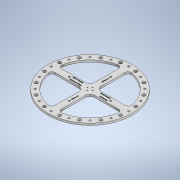
# Autodesk Inventor part: 24_Disco
Saved by Autodesk Inventor 2020.2 (Build 242310000, 310)
## iProperties
Created: 2019-11-29
Part Number: 24_Disco
Material: Generico
Document SubType Name: Modeling
Designer: socci
Density: 1 g/cm^3
Appearance: Default
Author: socci
Autodesk Inventor part; units mm, degrees
(part 1 of 3)
ref_plane "YZ Plane" through (0, 0, 0) normal (1, 0, 0) x (0, 1, 0)
ref_plane "XZ Plane" through (0, 0, 0) normal (0, 1, 0) x (-1, 0, 0)
ref_plane "XY Plane" through (0, 0, 0) normal (0, 0, 1) x (1, 0, 0)
sketch "Schizzo1" plane through (0, 0, 0) normal (0, 1, 0) x (-1, 0, 0)
  circle A0 centre (0, 0) radius 130
  line L0 (0, 130) -> (0, -130)
  line L1 (130, 0) -> (-130, 0)
  line L2 (10, 97.9796) -> (10, 23.6854)
  line L3 (97.9796, 10) -> (23.6854, 10)
  arc A1 (16.045, 13.5484) -> (13.5484, 16.045) centre (0, 0) ccw
  arc A2 (107.7775, 22) -> (22, 107.7775) centre (0, 0) ccw
  arc A3 (22, 107.7775) -> (10, 97.9796) centre (20, 97.9796) ccw
  arc A4 (10, 23.6854) -> (13.5484, 16.045) centre (20, 23.6854) ccw
  arc A5 (16.045, 13.5484) -> (23.6854, 10) centre (23.6854, 20) ccw
  arc A6 (97.9796, 10) -> (107.7775, 22) centre (97.9796, 20) ccw
  arc A7 (-13.5484, 16.045) -> (-10, 23.6854) centre (-20, 23.6854) ccw
  arc A8 (-13.5484, 16.045) -> (-16.045, 13.5484) centre (0, 0) ccw
  arc A9 (-23.6854, 10) -> (-16.045, 13.5484) centre (-23.6854, 20) ccw
  line L4 (-10, 97.9796) -> (-10, 23.6854)
  line L5 (-97.9796, 10) -> (-23.6854, 10)
  arc A10 (-107.7775, 22) -> (-97.9796, 10) centre (-97.9796, 20) ccw
  arc A11 (-22, 107.7775) -> (-107.7775, 22) centre (0, 0) ccw
  arc A12 (-10, 97.9796) -> (-22, 107.7775) centre (-20, 97.9796) ccw
  arc A13 (-16.045, -13.5484) -> (-23.6854, -10) centre (-23.6854, -20) ccw
  arc A14 (-16.045, -13.5484) -> (-13.5484, -16.045) centre (0, 0) ccw
  arc A15 (-10, -23.6854) -> (-13.5484, -16.045) centre (-20, -23.6854) ccw
  line L6 (-97.9796, -10) -> (-23.6854, -10)
  line L7 (-10, -97.9796) -> (-10, -23.6854)
  arc A16 (-22, -107.7775) -> (-10, -97.9796) centre (-20, -97.9796) ccw
  arc A17 (-107.7775, -22) -> (-22, -107.7775) centre (0, 0) ccw
  arc A18 (-97.9796, -10) -> (-107.7775, -22) centre (-97.9796, -20) ccw
  arc A19 (13.5484, -16.045) -> (10, -23.6854) centre (20, -23.6854) ccw
  arc A20 (13.5484, -16.045) -> (16.045, -13.5484) centre (0, 0) ccw
  arc A21 (23.6854, -10) -> (16.045, -13.5484) centre (23.6854, -20) ccw
  line L8 (10, -97.9796) -> (10, -23.6854)
  line L9 (97.9796, -10) -> (23.6854, -10)
  arc A22 (107.7775, -22) -> (97.9796, -10) centre (97.9796, -20) ccw
  arc A23 (22, -107.7775) -> (107.7775, -22) centre (0, 0) ccw
  arc A24 (10, -97.9796) -> (22, -107.7775) centre (20, -97.9796) ccw
  point P0 (18.4662, 10)
  point P1 (10, 18.4662)
  point P2 (109.5445, 10)
  point P3 (10, 109.5445)
  point P4 (-10, 18.4662)
  point P5 (-18.4662, 10)
  point P6 (-10, 109.5445)
  point P7 (-109.5445, 10)
  point P8 (-18.4662, -10)
  point P9 (-10, -18.4662)
  point P10 (-109.5445, -10)
  point P11 (-10, -109.5445)
  point P12 (10, -18.4662)
  point P13 (18.4662, -10)
  point P14 (10, -109.5445)
  point P15 (109.5445, -10)
  dimension "d0" = 260
  dimension "d2" = 10
  dimension "d5" = 10
  dimension "d7" = 10
  dimension "d10" = 360
  constraints: 68 point on circle, 25 centre point, 20 end point, 16 point on line, 8 tangent, 7 coincident, 3 equal radius, 2 parallel, 1 vertical, 107 other
  measures "d0" diameter of A0
  measures "d2" distance between parallel lines of L0 L2
  measures "d5" distance between parallel lines of L1 L3
  measures "d7" radius of A3
extrude "Estrusione1" add sketch "Schizzo1" along normal blind 6
sketch "Schizzo2" plane through (0, 6, 0) normal (0, 1, 0) x (1, 0, 0)
  line L0 (0, 0) -> (0, -8)
  line L1 (0, 0) -> (8, 0) construction
  point P0 (8, 0)
  point P1 (0, 8)
  point P2 (-8, 0)
  dimension "d14" = 8
  dimension "d15" = 90
  dimension "d18" = 360
  constraints: 4 end point, 1 coincident, 1 horizontal, 1 perpendicular, 1 vertical, 5 other
  measures "d14" distance of L0.start L0.end
  measures "d15" angle of L0 L1
hole "Foro1" at (0, 6, 8) at (0, 6, -8) at (8, 6, 0) at (-8, 6, 0) direction (0, -1, 0) diameter 3 end through all
sketch "Schizzo3" plane through (0, 6, 0) normal (0, 1, 0) x (1, 0, 0)
  line L0 (0, -110) -> (0, -130)
  circle A0 centre (0, 0) radius 130 projected
  line L1 (42.0952, -101.6267) -> (49.7488, -120.1043)
  line L2 (77.7817, -77.7817) -> (91.9239, -91.9239)
  line L3 (101.6267, -42.0952) -> (120.1043, -49.7488)
  line L4 (110, 0) -> (130, 0)
  line L5 (101.6267, 42.0952) -> (120.1043, 49.7488)
  line L6 (77.7817, 77.7817) -> (91.9239, 91.9239)
  line L7 (42.0952, 101.6267) -> (49.7488, 120.1043)
  line L8 (0, 110) -> (0, 130)
  line L9 (-42.0952, 101.6267) -> (-49.7488, 120.1043)
  line L10 (-77.7817, 77.7817) -> (-91.9239, 91.9239)
  line L11 (-101.6267, 42.0952) -> (-120.1043, 49.7488)
  line L12 (-110, 0) -> (-130, 0)
  line L13 (-101.6267, -42.0952) -> (-120.1043, -49.7488)
  line L14 (-77.7817, -77.7817) -> (-91.9239, -91.9239)
  line L15 (-42.0952, -101.6267) -> (-49.7488, -120.1043)
  circle A1 centre (0, -8) radius 1.5 projected
  line L16 (0, -8) -> (0, -120)
  point P0 (45.922, -110.8655)
  point P1 (84.8528, -84.8528)
  point P2 (110.8655, -45.922)
  point P3 (120, 0)
  point P4 (110.8655, 45.922)
  point P5 (84.8528, 84.8528)
  point P6 (45.922, 110.8655)
  point P7 (0, 120)
  point P8 (-45.922, 110.8655)
  point P9 (-84.8528, 84.8528)
  point P10 (-110.8655, 45.922)
  point P11 (-120, 0)
  point P12 (-110.8655, -45.922)
  point P13 (-84.8528, -84.8528)
  point P14 (-45.922, -110.8655)
  point P15 (0, -64)
  point P16 (64, 0)
  point P17 (0, 64)
  point P18 (-64, 0)
  dimension "d29" = 360
  dimension "d33" = 360
  constraints: 34 end point, 4 coincident, 2 midpoint, 2 vertical, 1 vertical alignment, 87 other
hole "Foro2" at (0, 6, 120) at (45.922, 6, 110.8655) at (84.8528, 6, 84.8528) at (110.8655, 6, 45.922) at (120, 6, 0) at (110.8655, 6, -45.922) at (84.8528, 6, -84.8528) at (45.922, 6, -110.8655) at (0, 6, -120) at (-45.922, 6, -110.8655) at (-84.8528, 6, -84.8528) at (-110.8655, 6, -45.922) at (-120, 6, 0) at (-110.8655, 6, 45.922) at (-84.8528, 6, 84.8528) at (-45.922, 6, 110.8655) at (0, 6, 64) at (64, 6, 0) at (0, 6, -64) at (-64, 6, 0) direction (0, -1, 0) diameter 6 end through all
sketch "Schizzo4" plane through (0, 6, 0) normal (0, 1, 0) x (1, 0, 0)
  circle A0 centre (0, -120) radius 3 projected
  circle A1 centre (45.922, -110.8655) radius 3 projected
  arc A2 (0, -120) -> (45.922, -110.8655) centre (0, 0) ccw
  point P0 (23.4108, -117.6942)
  point P1 (66.6684, -99.7764)
  point P2 (99.7764, -66.6684)
  point P3 (117.6942, -23.4108)
  point P4 (117.6942, 23.4108)
  point P5 (99.7764, 66.6684)
  point P6 (66.6684, 99.7764)
  point P7 (23.4108, 117.6942)
  point P8 (-23.4108, 117.6942)
  point P9 (-66.6684, 99.7764)
  point P10 (-99.7764, 66.6684)
  point P11 (-117.6942, 23.4108)
  point P12 (-117.6942, -23.4108)
  point P13 (-99.7764, -66.6684)
  point P14 (-66.6684, -99.7764)
  point P15 (-23.4108, -117.6942)
  dimension "d44" = 360
  constraints: 3 point on circle, 1 centre point, 1 coincident, 17 other
hole "Foro3" at (23.4108, 6, 117.6942) at (66.6684, 6, 99.7764) at (99.7764, 6, 66.6684) at (117.6942, 6, 23.4108) at (117.6942, 6, -23.4108) at (99.7764, 6, -66.6684) at (66.6684, 6, -99.7764) at (23.4108, 6, -117.6942) at (-23.4108, 6, -117.6942) at (-66.6684, 6, -99.7764) at (-99.7764, 6, -66.6684) at (-117.6942, 6, -23.4108) at (-117.6942, 6, 23.4108) at (-99.7764, 6, 66.6684) at (-66.6684, 6, 99.7764) at (-23.4108, 6, 117.6942) direction (0, -1, 0) diameter 10 end through all
sketch "Schizzo5" plane through (0, 6, 0) normal (0, 1, 0) x (1, 0, 0)
  line L0 (-58, 7.2418) -> (-17.0463, 7.2418) construction
  line L1 (-17.0463, 7.2418) -> (-17.0463, -7.2418) construction
  line L2 (-17.0463, -7.2418) -> (-58, -7.2418) construction
  line L3 (-58, -7.2418) -> (-58, 7.2418) construction
  line L4 (-182, 0) -> (182, 0) projected
  circle A0 centre (-64, 0) radius 3 projected
  circle A1 centre (-64, 0) radius 6 construction
  line L5 (22.5156, 7.2418) -> (58, 7.2418) construction
  line L6 (58, 7.2418) -> (58, -7.2418) construction
  line L7 (58, -7.2418) -> (22.5156, -7.2418) construction
  line L8 (22.5156, -7.2418) -> (22.5156, 7.2418) construction
  circle A2 centre (64, 0) radius 3 projected
  circle A3 centre (64, 0) radius 6 construction
  circle A4 centre (0, 0) radius 12.5 construction
  line L9 (1.948, -32.3891) -> (1.948, -57.7549) construction
  line L10 (1.948, -57.7549) -> (-2.4438, -57.7549) construction
  line L11 (-2.4438, -57.7549) -> (-2.4438, -32.3891) construction
  line L12 (-2.4438, -32.3891) -> (1.948, -32.3891) construction
  line L13 (0, 182) -> (0, -182) projected
  circle A5 centre (0, -64) radius 3 projected
  line L14 (1.948, 57.7549) -> (1.948, 27.0589) construction
  line L15 (1.948, 27.0589) -> (-2.4438, 27.0589) construction
  line L16 (-2.4438, 27.0589) -> (-2.4438, 57.7549) construction
  line L17 (-2.4438, 57.7549) -> (1.948, 57.7549) construction
  circle A6 centre (0, 64) radius 3 projected
  circle A7 centre (0, -64) radius 6.25 construction
  circle A8 centre (0, 64) radius 6.25 construction
  line L18 (-58.0198, 4.0382) -> (-56.9922, 7.0862)
  line L19 (-56.9922, 7.0862) -> (-56.4933, 7.0862)
  line L20 (-56.4933, 7.0862) -> (-55.4658, 4.0382)
  line L21 (-55.4658, 4.0382) -> (-55.8931, 4.0382)
  line L22 (-55.8931, 4.0382) -> (-56.1697, 4.8903)
  line L23 (-56.1697, 4.8903) -> (-57.3331, 4.8903)
  line L24 (-57.3331, 4.8903) -> (-57.6097, 4.0382)
  line L25 (-57.6097, 4.0382) -> (-58.0198, 4.0382)
  line L26 (-56.2809, 5.2361) -> (-56.7526, 6.6712)
  line L27 (-56.7526, 6.6712) -> (-57.2219, 5.2361)
  line L28 (-57.2219, 5.2361) -> (-56.2809, 5.2361)
  line L29 (-54.8137, 4.0382) -> (-55.199, 4.0382)
  line L30 (-55.199, 4.0382) -> (-55.199, 7.222)
  line L31 (-55.199, 7.222) -> (-54.8137, 7.222)
  line L32 (-54.8137, 7.222) -> (-54.8137, 4.0382)
  line L33 (-53.0451, 6.8515) -> (-53.0649, 6.8515)
  spline S0 degree 2 poles (-53.0649, 6.8515) (-53.1168, 6.8713) (-53.3094, 6.9059) (-53.386, 6.9059) knots 0 0 0 1 2 2 2
  spline S1 degree 2 poles (-53.386, 6.9059) (-53.6281, 6.9059) (-53.8356, 6.6885) (-53.8356, 6.402) knots 0 0 0 1 2 2 2
  line L34 (-53.8356, 6.402) -> (-53.8356, 6.3254)
  line L35 (-53.8356, 6.3254) -> (-53.1983, 6.3254)
  line L36 (-53.1983, 6.3254) -> (-53.1983, 6.0068)
  line L37 (-53.1983, 6.0068) -> (-53.8232, 6.0068)
  line L38 (-53.8232, 6.0068) -> (-53.8232, 4.0382)
  line L39 (-53.8232, 4.0382) -> (-54.2085, 4.0382)
  line L40 (-54.2085, 4.0382) -> (-54.2085, 6.0068)
  line L41 (-54.2085, 6.0068) -> (-54.4679, 6.0068)
  line L42 (-54.4679, 6.0068) -> (-54.4679, 6.3254)
  line L43 (-54.4679, 6.3254) -> (-54.2085, 6.3254)
  line L44 (-54.2085, 6.3254) -> (-54.2085, 6.402)
  spline S2 degree 2 poles (-54.2085, 6.402) (-54.2085, 6.812) (-53.8109, 7.2418) (-53.4404, 7.2418) knots 0 0 0 1 2 2 2
  spline S3 degree 2 poles (-53.4404, 7.2418) (-53.3341, 7.2418) (-53.1291, 7.2196) (-53.0451, 7.2047) knots 0 0 0 1 2 2 2
  line L45 (-53.0451, 7.2047) -> (-53.0451, 6.8515)
  spline S4 degree 2 poles (-51.6397, 4.2802) (-51.6866, 4.2457) (-51.8447, 4.1222) (-51.9188, 4.0851) knots 0 0 0 1 2 2 2
  spline S5 degree 2 poles (-51.9188, 4.0851) (-52.0201, 4.0308) (-52.2103, 3.974) (-52.3832, 3.974) knots 0 0 0 1 2 2 2
  spline S6 degree 2 poles (-52.3832, 3.974) (-52.524, 3.974) (-52.7784, 4.0802) (-52.8747, 4.1765) knots 0 0 0 1 2 2 2
  spline S7 degree 2 poles (-52.8747, 4.1765) (-52.9661, 4.2704) (-53.0773, 4.547) (-53.0773, 4.7001) knots 0 0 0 1 2 2 2
  spline S8 degree 2 poles (-53.0773, 4.7001) (-53.0773, 4.9373) (-52.8772, 5.2732) (-52.6598, 5.3695) knots 0 0 0 1 2 2 2
  spline S9 degree 2 poles (-52.6598, 5.3695) (-52.4672, 5.4584) (-51.9435, 5.5251) (-51.6397, 5.5424) knots 0 0 0 1 2 2 2
  line L46 (-51.6397, 5.5424) -> (-51.6397, 5.6165)
  spline S10 degree 2 poles (-51.6397, 5.6165) (-51.6397, 5.7499) (-51.7212, 5.9154) (-51.7953, 5.9623) knots 0 0 0 1 2 2 2
  spline S11 degree 2 poles (-51.7953, 5.9623) (-51.8694, 6.0093) (-52.0818, 6.0389) (-52.1955, 6.0389) knots 0 0 0 1 2 2 2
  spline S12 degree 2 poles (-52.1955, 6.0389) (-52.3288, 6.0389) (-52.6895, 5.9599) (-52.8698, 5.8833) knots 0 0 0 1 2 2 2
  line L47 (-52.8698, 5.8833) -> (-52.892, 5.8833)
  line L48 (-52.892, 5.8833) -> (-52.892, 6.276)
  spline S13 degree 2 poles (-52.892, 6.276) (-52.7858, 6.3057) (-52.3881, 6.3798) (-52.193, 6.3798) knots 0 0 0 1 2 2 2
  spline S14 degree 2 poles (-52.193, 6.3798) (-51.9559, 6.3798) (-51.6323, 6.3057) (-51.5039, 6.2093) knots 0 0 0 1 2 2 2
  spline S15 degree 2 poles (-51.5039, 6.2093) (-51.3779, 6.1155) (-51.2544, 5.8166) (-51.2544, 5.6017) knots 0 0 0 1 2 2 2
  line L49 (-51.2544, 5.6017) -> (-51.2544, 4.0382)
  line L50 (-51.2544, 4.0382) -> (-51.6397, 4.0382)
  line L51 (-51.6397, 4.0382) -> (-51.6397, 4.2802)
  line L52 (-51.6397, 4.6013) -> (-51.6397, 5.2361)
  spline S16 degree 2 poles (-51.6397, 5.2361) (-51.778, 5.2238) (-52.1955, 5.1818) (-52.3264, 5.1423) knots 0 0 0 1 2 2 2
  spline S17 degree 2 poles (-52.3264, 5.1423) (-52.4795, 5.0954) (-52.6796, 4.9002) (-52.6796, 4.7273) knots 0 0 0 1 2 2 2
  spline S18 degree 2 poles (-52.6796, 4.7273) (-52.6796, 4.5297) (-52.4573, 4.3296) (-52.2449, 4.3296) knots 0 0 0 1 2 2 2
  spline S19 degree 2 poles (-52.2449, 4.3296) (-52.0646, 4.3296) (-51.7681, 4.4853) (-51.6397, 4.6013) knots 0 0 0 1 2 2 2
  line L53 (-48.9178, 4.0382) -> (-49.3031, 4.0382)
  line L54 (-49.3031, 4.0382) -> (-49.3031, 5.3424)
  spline S20 degree 2 poles (-49.3031, 5.3424) (-49.3031, 5.5004) (-49.3327, 5.7721) (-49.3772, 5.8536) knots 0 0 0 1 2 2 2
  spline S21 degree 2 poles (-49.3772, 5.8536) (-49.4241, 5.9401) (-49.5921, 6.0241) (-49.7353, 6.0241) knots 0 0 0 1 2 2 2
  spline S22 degree 2 poles (-49.7353, 6.0241) (-49.8786, 6.0241) (-50.1824, 5.8709) (-50.3281, 5.7474) knots 0 0 0 1 2 2 2
  line L55 (-50.3281, 5.7474) -> (-50.3281, 4.0382)
  line L56 (-50.3281, 4.0382) -> (-50.7135, 4.0382)
  line L57 (-50.7135, 4.0382) -> (-50.7135, 6.3254)
  line L58 (-50.7135, 6.3254) -> (-50.3281, 6.3254)
  line L59 (-50.3281, 6.3254) -> (-50.3281, 6.071)
  spline S23 degree 2 poles (-50.3281, 6.071) (-50.1552, 6.2266) (-49.8218, 6.3896) (-49.6341, 6.3896) knots 0 0 0 1 2 2 2
  spline S24 degree 2 poles (-49.6341, 6.3896) (-49.2981, 6.3896) (-48.9178, 5.945) (-48.9178, 5.5227) knots 0 0 0 1 2 2 2
  line L60 (-48.9178, 5.5227) -> (-48.9178, 4.0382)
  spline S25 degree 2 poles (-46.4971, 5.1818) (-46.4971, 4.6038) (-47.0529, 3.974) (-47.5173, 3.974) knots 0 0 0 1 2 2 2
  spline S26 degree 2 poles (-47.5173, 3.974) (-47.994, 3.974) (-48.5398, 4.6236) (-48.5398, 5.1818) knots 0 0 0 1 2 2 2
  spline S27 degree 2 poles (-48.5398, 5.1818) (-48.5398, 5.7548) (-47.9767, 6.3896) (-47.5173, 6.3896) knots 0 0 0 1 2 2 2
  spline S28 degree 2 poles (-47.5173, 6.3896) (-47.0529, 6.3896) (-46.4971, 5.7573) (-46.4971, 5.1818) knots 0 0 0 1 2 2 2
  spline S29 degree 2 poles (-46.8948, 5.1818) (-46.8948, 5.6264) (-47.2184, 6.0587) (-47.5173, 6.0587) knots 0 0 0 1 2 2 2
  spline S30 degree 2 poles (-47.5173, 6.0587) (-47.8161, 6.0587) (-48.1422, 5.6264) (-48.1422, 5.1818) knots 0 0 0 1 2 2 2
  spline S31 degree 2 poles (-48.1422, 5.1818) (-48.1422, 4.7495) (-47.8161, 4.3049) (-47.5173, 4.3049) knots 0 0 0 1 2 2 2
  spline S32 degree 2 poles (-47.5173, 4.3049) (-47.2208, 4.3049) (-46.8948, 4.7421) (-46.8948, 5.1818) knots 0 0 0 1 2 2 2
  line L61 (-44.7632, 4.0382) -> (-44.7632, 7.0862)
  line L62 (-44.7632, 7.0862) -> (-42.8563, 7.0862)
  line L63 (-42.8563, 7.0862) -> (-42.8563, 6.7256)
  line L64 (-42.8563, 6.7256) -> (-44.3581, 6.7256)
  line L65 (-44.3581, 6.7256) -> (-44.3581, 5.8907)
  line L66 (-44.3581, 5.8907) -> (-42.9576, 5.8907)
  line L67 (-42.9576, 5.8907) -> (-42.9576, 5.5301)
  line L68 (-42.9576, 5.5301) -> (-44.3581, 5.5301)
  line L69 (-44.3581, 5.5301) -> (-44.3581, 4.3988)
  line L70 (-44.3581, 4.3988) -> (-42.8563, 4.3988)
  line L71 (-42.8563, 4.3988) -> (-42.8563, 4.0382)
  line L72 (-42.8563, 4.0382) -> (-44.7632, 4.0382)
  line L73 (-39.8479, 4.0382) -> (-39.8479, 5.3621)
  spline S33 degree 2 poles (-39.8479, 5.3621) (-39.8479, 5.5202) (-39.8726, 5.7894) (-39.9121, 5.8635) knots 0 0 0 1 2 2 2
  spline S34 degree 2 poles (-39.9121, 5.8635) (-39.9516, 5.945) (-40.1023, 6.0241) (-40.2332, 6.0241) knots 0 0 0 1 2 2 2
  spline S35 degree 2 poles (-40.2332, 6.0241) (-40.3517, 6.0241) (-40.6234, 5.8783) (-40.7667, 5.74) knots 0 0 0 1 2 2 2
  spline S36 degree 2 poles (-40.7667, 5.74) (-40.7642, 5.7054) (-40.7593, 5.6091) (-40.7593, 5.5449) knots 0 0 0 1 2 2 2
  line L74 (-40.7593, 5.5449) -> (-40.7593, 4.0382)
  line L75 (-40.7593, 4.0382) -> (-41.1446, 4.0382)
  line L76 (-41.1446, 4.0382) -> (-41.1446, 5.3621)
  spline S37 degree 2 poles (-41.1446, 5.3621) (-41.1446, 5.5202) (-41.1693, 5.7894) (-41.2088, 5.8635) knots 0 0 0 1 2 2 2
  spline S38 degree 2 poles (-41.2088, 5.8635) (-41.2483, 5.945) (-41.399, 6.0241) (-41.5299, 6.0241) knots 0 0 0 1 2 2 2
  spline S39 degree 2 poles (-41.5299, 6.0241) (-41.6534, 6.0241) (-41.9276, 5.8685) (-42.056, 5.7474) knots 0 0 0 1 2 2 2
  line L77 (-42.056, 5.7474) -> (-42.056, 4.0382)
  line L78 (-42.056, 4.0382) -> (-42.4414, 4.0382)
  line L79 (-42.4414, 4.0382) -> (-42.4414, 6.3254)
  line L80 (-42.4414, 6.3254) -> (-42.056, 6.3254)
  line L81 (-42.056, 6.3254) -> (-42.056, 6.0735)
  spline S40 degree 2 poles (-42.056, 6.0735) (-41.9054, 6.2241) (-41.609, 6.3896) (-41.4311, 6.3896) knots 0 0 0 1 2 2 2
  spline S41 degree 2 poles (-41.4311, 6.3896) (-41.2286, 6.3896) (-40.9149, 6.2044) (-40.8334, 5.9944) knots 0 0 0 1 2 2 2
  spline S42 degree 2 poles (-40.8334, 5.9944) (-40.658, 6.1896) (-40.327, 6.3896) (-40.1344, 6.3896) knots 0 0 0 1 2 2 2
  spline S43 degree 2 poles (-40.1344, 6.3896) (-39.9862, 6.3896) (-39.7441, 6.2982) (-39.6552, 6.1945) knots 0 0 0 1 2 2 2
  spline S44 degree 2 poles (-39.6552, 6.1945) (-39.5638, 6.0908) (-39.4625, 5.7795) (-39.4625, 5.5449) knots 0 0 0 1 2 2 2
  line L82 (-39.4625, 5.5449) -> (-39.4625, 4.0382)
  line L83 (-39.4625, 4.0382) -> (-39.8479, 4.0382)
  spline S45 degree 2 poles (-37.6471, 4.2802) (-37.694, 4.2457) (-37.8521, 4.1222) (-37.9262, 4.0851) knots 0 0 0 1 2 2 2
  spline S46 degree 2 poles (-37.9262, 4.0851) (-38.0274, 4.0308) (-38.2176, 3.974) (-38.3905, 3.974) knots 0 0 0 1 2 2 2
  spline S47 degree 2 poles (-38.3905, 3.974) (-38.5313, 3.974) (-38.7857, 4.0802) (-38.8821, 4.1765) knots 0 0 0 1 2 2 2
  spline S48 degree 2 poles (-38.8821, 4.1765) (-38.9735, 4.2704) (-39.0846, 4.547) (-39.0846, 4.7001) knots 0 0 0 1 2 2 2
  spline S49 degree 2 poles (-39.0846, 4.7001) (-39.0846, 4.9373) (-38.8845, 5.2732) (-38.6672, 5.3695) knots 0 0 0 1 2 2 2
  spline S50 degree 2 poles (-38.6672, 5.3695) (-38.4745, 5.4584) (-37.9509, 5.5251) (-37.6471, 5.5424) knots 0 0 0 1 2 2 2
  line L84 (-37.6471, 5.5424) -> (-37.6471, 5.6165)
  spline S51 degree 2 poles (-37.6471, 5.6165) (-37.6471, 5.7499) (-37.7286, 5.9154) (-37.8027, 5.9623) knots 0 0 0 1 2 2 2
  spline S52 degree 2 poles (-37.8027, 5.9623) (-37.8768, 6.0093) (-38.0892, 6.0389) (-38.2028, 6.0389) knots 0 0 0 1 2 2 2
  spline S53 degree 2 poles (-38.2028, 6.0389) (-38.3362, 6.0389) (-38.6968, 5.9599) (-38.8771, 5.8833) knots 0 0 0 1 2 2 2
  line L85 (-38.8771, 5.8833) -> (-38.8994, 5.8833)
  line L86 (-38.8994, 5.8833) -> (-38.8994, 6.276)
  spline S54 degree 2 poles (-38.8994, 6.276) (-38.7932, 6.3057) (-38.3955, 6.3798) (-38.2003, 6.3798) knots 0 0 0 1 2 2 2
  spline S55 degree 2 poles (-38.2003, 6.3798) (-37.9632, 6.3798) (-37.6397, 6.3057) (-37.5112, 6.2093) knots 0 0 0 1 2 2 2
  spline S56 degree 2 poles (-37.5112, 6.2093) (-37.3852, 6.1155) (-37.2617, 5.8166) (-37.2617, 5.6017) knots 0 0 0 1 2 2 2
  line L87 (-37.2617, 5.6017) -> (-37.2617, 4.0382)
  line L88 (-37.2617, 4.0382) -> (-37.6471, 4.0382)
  line L89 (-37.6471, 4.0382) -> (-37.6471, 4.2802)
  line L90 (-37.6471, 4.6013) -> (-37.6471, 5.2361)
  spline S57 degree 2 poles (-37.6471, 5.2361) (-37.7854, 5.2238) (-38.2028, 5.1818) (-38.3337, 5.1423) knots 0 0 0 1 2 2 2
  spline S58 degree 2 poles (-38.3337, 5.1423) (-38.4869, 5.0954) (-38.6869, 4.9002) (-38.6869, 4.7273) knots 0 0 0 1 2 2 2
  spline S59 degree 2 poles (-38.6869, 4.7273) (-38.6869, 4.5297) (-38.4646, 4.3296) (-38.2522, 4.3296) knots 0 0 0 1 2 2 2
  spline S60 degree 2 poles (-38.2522, 4.3296) (-38.0719, 4.3296) (-37.7755, 4.4853) (-37.6471, 4.6013) knots 0 0 0 1 2 2 2
  line L91 (-34.9251, 4.0382) -> (-35.3104, 4.0382)
  line L92 (-35.3104, 4.0382) -> (-35.3104, 5.3424)
  spline S61 degree 2 poles (-35.3104, 5.3424) (-35.3104, 5.5004) (-35.3401, 5.7721) (-35.3845, 5.8536) knots 0 0 0 1 2 2 2
  spline S62 degree 2 poles (-35.3845, 5.8536) (-35.4315, 5.9401) (-35.5994, 6.0241) (-35.7427, 6.0241) knots 0 0 0 1 2 2 2
  spline S63 degree 2 poles (-35.7427, 6.0241) (-35.8859, 6.0241) (-36.1898, 5.8709) (-36.3355, 5.7474) knots 0 0 0 1 2 2 2
  line L93 (-36.3355, 5.7474) -> (-36.3355, 4.0382)
  line L94 (-36.3355, 4.0382) -> (-36.7208, 4.0382)
  line L95 (-36.7208, 4.0382) -> (-36.7208, 6.3254)
  line L96 (-36.7208, 6.3254) -> (-36.3355, 6.3254)
  line L97 (-36.3355, 6.3254) -> (-36.3355, 6.071)
  spline S64 degree 2 poles (-36.3355, 6.071) (-36.1626, 6.2266) (-35.8291, 6.3896) (-35.6414, 6.3896) knots 0 0 0 1 2 2 2
  spline S65 degree 2 poles (-35.6414, 6.3896) (-35.3055, 6.3896) (-34.9251, 5.945) (-34.9251, 5.5227) knots 0 0 0 1 2 2 2
  line L98 (-34.9251, 5.5227) -> (-34.9251, 4.0382)
  line L99 (-32.6058, 4.0382) -> (-32.9911, 4.0382)
  line L100 (-32.9911, 4.0382) -> (-32.9911, 4.2901)
  spline S66 degree 2 poles (-32.9911, 4.2901) (-33.1689, 4.1345) (-33.4876, 3.974) (-33.6852, 3.974) knots 0 0 0 1 2 2 2
  spline S67 degree 2 poles (-33.6852, 3.974) (-33.8334, 3.974) (-34.0977, 4.0728) (-34.194, 4.179) knots 0 0 0 1 2 2 2
  spline S68 degree 2 poles (-34.194, 4.179) (-34.2928, 4.2852) (-34.4015, 4.6088) (-34.4015, 4.8409) knots 0 0 0 1 2 2 2
  line L101 (-34.4015, 4.8409) -> (-34.4015, 6.3254)
  line L102 (-34.4015, 6.3254) -> (-34.0161, 6.3254)
  line L103 (-34.0161, 6.3254) -> (-34.0161, 5.0213)
  spline S69 degree 2 poles (-34.0161, 5.0213) (-34.0161, 4.8385) (-33.989, 4.5989) (-33.942, 4.51) knots 0 0 0 1 2 2 2
  spline S70 degree 2 poles (-33.942, 4.51) (-33.8951, 4.421) (-33.7346, 4.3395) (-33.5839, 4.3395) knots 0 0 0 1 2 2 2
  spline S71 degree 2 poles (-33.5839, 4.3395) (-33.4431, 4.3395) (-33.1245, 4.5001) (-32.9911, 4.6162) knots 0 0 0 1 2 2 2
  line L104 (-32.9911, 4.6162) -> (-32.9911, 6.3254)
  line L105 (-32.9911, 6.3254) -> (-32.6058, 6.3254)
  line L106 (-32.6058, 6.3254) -> (-32.6058, 4.0382)
  spline S72 degree 2 poles (-31.0546, 3.9863) (-31.6029, 3.9863) (-32.2056, 4.6013) (-32.2056, 5.1695) knots 0 0 0 1 2 2 2
  spline S73 degree 2 poles (-32.2056, 5.1695) (-32.2056, 5.7277) (-31.6202, 6.3896) (-31.1485, 6.3896) knots 0 0 0 1 2 2 2
  spline S74 degree 2 poles (-31.1485, 6.3896) (-30.936, 6.3896) (-30.6075, 6.2661) (-30.4865, 6.1352) knots 0 0 0 1 2 2 2
  spline S75 degree 2 poles (-30.4865, 6.1352) (-30.363, 6.0043) (-30.2321, 5.6264) (-30.2321, 5.3522) knots 0 0 0 1 2 2 2
  line L107 (-30.2321, 5.3522) -> (-30.2321, 5.1423)
  line L108 (-30.2321, 5.1423) -> (-31.8154, 5.1423)
  spline S76 degree 2 poles (-31.8154, 5.1423) (-31.8154, 4.7446) (-31.4152, 4.3222) (-31.0595, 4.3222) knots 0 0 0 1 2 2 2
  spline S77 degree 2 poles (-31.0595, 4.3222) (-30.9336, 4.3222) (-30.689, 4.379) (-30.5902, 4.4235) knots 0 0 0 1 2 2 2
  spline S78 degree 2 poles (-30.5902, 4.4235) (-30.4865, 4.4729) (-30.3432, 4.5594) (-30.2963, 4.5989) knots 0 0 0 1 2 2 2
  line L109 (-30.2963, 4.5989) -> (-30.2741, 4.5989)
  line L110 (-30.2741, 4.5989) -> (-30.2741, 4.179)
  spline S79 degree 2 poles (-30.2741, 4.179) (-30.3408, 4.1518) (-30.5433, 4.0728) (-30.6223, 4.0505) knots 0 0 0 1 2 2 2
  spline S80 degree 2 poles (-30.6223, 4.0505) (-30.7335, 4.0184) (-30.9163, 3.9863) (-31.0546, 3.9863) knots 0 0 0 1 2 2 2
  spline S81 degree 2 poles (-30.6075, 5.4362) (-30.6125, 5.5918) (-30.6767, 5.8191) (-30.7384, 5.8956) knots 0 0 0 1 2 2 2
  spline S82 degree 2 poles (-30.7384, 5.8956) (-30.8051, 5.9821) (-31.0151, 6.0735) (-31.1707, 6.0735) knots 0 0 0 1 2 2 2
  spline S83 degree 2 poles (-31.1707, 6.0735) (-31.3238, 6.0735) (-31.5387, 5.9821) (-31.6276, 5.8932) knots 0 0 0 1 2 2 2
  spline S84 degree 2 poles (-31.6276, 5.8932) (-31.7141, 5.8018) (-31.803, 5.5819) (-31.8154, 5.4362) knots 0 0 0 1 2 2 2
  line L111 (-31.8154, 5.4362) -> (-30.6075, 5.4362)
  line L112 (-29.4491, 4.0382) -> (-29.8344, 4.0382)
  line L113 (-29.8344, 4.0382) -> (-29.8344, 7.222)
  line L114 (-29.8344, 7.222) -> (-29.4491, 7.222)
  line L115 (-29.4491, 7.222) -> (-29.4491, 4.0382)
  spline S85 degree 2 poles (-27.8905, 3.9863) (-28.4388, 3.9863) (-29.0415, 4.6013) (-29.0415, 5.1695) knots 0 0 0 1 2 2 2
  spline S86 degree 2 poles (-29.0415, 5.1695) (-29.0415, 5.7277) (-28.4561, 6.3896) (-27.9844, 6.3896) knots 0 0 0 1 2 2 2
  spline S87 degree 2 poles (-27.9844, 6.3896) (-27.7719, 6.3896) (-27.4434, 6.2661) (-27.3224, 6.1352) knots 0 0 0 1 2 2 2
  spline S88 degree 2 poles (-27.3224, 6.1352) (-27.1989, 6.0043) (-27.068, 5.6264) (-27.068, 5.3522) knots 0 0 0 1 2 2 2
  line L116 (-27.068, 5.3522) -> (-27.068, 5.1423)
  line L117 (-27.068, 5.1423) -> (-28.6513, 5.1423)
  spline S89 degree 2 poles (-28.6513, 5.1423) (-28.6513, 4.7446) (-28.2511, 4.3222) (-27.8954, 4.3222) knots 0 0 0 1 2 2 2
  spline S90 degree 2 poles (-27.8954, 4.3222) (-27.7695, 4.3222) (-27.5249, 4.379) (-27.4261, 4.4235) knots 0 0 0 1 2 2 2
  spline S91 degree 2 poles (-27.4261, 4.4235) (-27.3224, 4.4729) (-27.1791, 4.5594) (-27.1322, 4.5989) knots 0 0 0 1 2 2 2
  line L118 (-27.1322, 4.5989) -> (-27.11, 4.5989)
  line L119 (-27.11, 4.5989) -> (-27.11, 4.179)
  spline S92 degree 2 poles (-27.11, 4.179) (-27.1767, 4.1518) (-27.3792, 4.0728) (-27.4582, 4.0505) knots 0 0 0 1 2 2 2
  spline S93 degree 2 poles (-27.4582, 4.0505) (-27.5694, 4.0184) (-27.7522, 3.9863) (-27.8905, 3.9863) knots 0 0 0 1 2 2 2
  spline S94 degree 2 poles (-27.4434, 5.4362) (-27.4484, 5.5918) (-27.5126, 5.8191) (-27.5743, 5.8956) knots 0 0 0 1 2 2 2
  spline S95 degree 2 poles (-27.5743, 5.8956) (-27.641, 5.9821) (-27.851, 6.0735) (-28.0066, 6.0735) knots 0 0 0 1 2 2 2
  spline S96 degree 2 poles (-28.0066, 6.0735) (-28.1597, 6.0735) (-28.3746, 5.9821) (-28.4635, 5.8932) knots 0 0 0 1 2 2 2
  spline S97 degree 2 poles (-28.4635, 5.8932) (-28.55, 5.8018) (-28.6389, 5.5819) (-28.6513, 5.4362) knots 0 0 0 1 2 2 2
  line L120 (-28.6513, 5.4362) -> (-27.4434, 5.4362)
  spline S98 degree 2 poles (-55.6238, -5.0626) (-55.6238, -5.2898) (-55.7967, -5.6381) (-55.94, -5.7517) knots 0 0 0 1 2 2 2
  spline S99 degree 2 poles (-55.94, -5.7517) (-56.1129, -5.8851) (-56.5056, -5.9987) (-56.8169, -5.9987) knots 0 0 0 1 2 2 2
  line L121 (-56.8169, -5.9987) -> (-57.6912, -5.9987)
  line L122 (-57.6912, -5.9987) -> (-57.6912, -2.9507)
  line L123 (-57.6912, -2.9507) -> (-56.8836, -2.9507)
  spline S100 degree 2 poles (-56.8836, -2.9507) (-56.5575, -2.9507) (-56.2315, -2.9927) (-56.0833, -3.0742) knots 0 0 0 1 2 2 2
  spline S101 degree 2 poles (-56.0833, -3.0742) (-55.9178, -3.1607) (-55.7671, -3.4447) (-55.7671, -3.6374) knots 0 0 0 1 2 2 2
  spline S102 degree 2 poles (-55.7671, -3.6374) (-55.7671, -3.8523) (-55.9943, -4.1931) (-56.1944, -4.2895) knots 0 0 0 1 2 2 2
  line L124 (-56.1944, -4.2895) -> (-56.1944, -4.3043)
  spline S103 degree 2 poles (-56.1944, -4.3043) (-55.9227, -4.3784) (-55.6238, -4.7711) (-55.6238, -5.0626) knots 0 0 0 1 2 2 2
  spline S104 degree 2 poles (-56.0462, -5.0799) (-56.0462, -4.907) (-56.145, -4.6847) (-56.2932, -4.6056) knots 0 0 0 1 2 2 2
  spline S105 degree 2 poles (-56.2932, -4.6056) (-56.3895, -4.5562) (-56.6168, -4.5266) (-56.8267, -4.5266) knots 0 0 0 1 2 2 2
  line L125 (-56.8267, -4.5266) -> (-57.2862, -4.5266)
  line L126 (-57.2862, -4.5266) -> (-57.2862, -5.6529)
  line L127 (-57.2862, -5.6529) -> (-56.9577, -5.6529)
  spline S106 degree 2 poles (-56.9577, -5.6529) (-56.6909, -5.6529) (-56.3846, -5.6035) (-56.266, -5.5245) knots 0 0 0 1 2 2 2
  spline S107 degree 2 poles (-56.266, -5.5245) (-56.1524, -5.443) (-56.0462, -5.2404) (-56.0462, -5.0799) knots 0 0 0 1 2 2 2
  spline S108 degree 2 poles (-56.1895, -3.6942) (-56.1895, -3.5855) (-56.2636, -3.4225) (-56.3451, -3.3756) knots 0 0 0 1 2 2 2
  spline S109 degree 2 poles (-56.3451, -3.3756) (-56.4439, -3.3212) (-56.6835, -3.2965) (-56.8984, -3.2965) knots 0 0 0 1 2 2 2
  line L128 (-56.8984, -3.2965) -> (-57.2862, -3.2965)
  line L129 (-57.2862, -3.2965) -> (-57.2862, -4.1882)
  line L130 (-57.2862, -4.1882) -> (-56.8267, -4.1882)
  spline S110 degree 2 poles (-56.8267, -4.1882) (-56.6366, -4.1882) (-56.4562, -4.1487) (-56.3599, -4.0869) knots 0 0 0 1 2 2 2
  spline S111 degree 2 poles (-56.3599, -4.0869) (-56.266, -4.0276) (-56.1895, -3.8375) (-56.1895, -3.6942) knots 0 0 0 1 2 2 2
  spline S112 degree 2 poles (-53.9763, -5.7567) (-54.0233, -5.7912) (-54.1814, -5.9147) (-54.2555, -5.9518) knots 0 0 0 1 2 2 2
  spline S113 degree 2 poles (-54.2555, -5.9518) (-54.3567, -6.0061) (-54.5469, -6.0629) (-54.7198, -6.0629) knots 0 0 0 1 2 2 2
  spline S114 degree 2 poles (-54.7198, -6.0629) (-54.8606, -6.0629) (-55.115, -5.9567) (-55.2114, -5.8604) knots 0 0 0 1 2 2 2
  spline S115 degree 2 poles (-55.2114, -5.8604) (-55.3027, -5.7665) (-55.4139, -5.4899) (-55.4139, -5.3368) knots 0 0 0 1 2 2 2
  spline S116 degree 2 poles (-55.4139, -5.3368) (-55.4139, -5.0996) (-55.2138, -4.7637) (-54.9965, -4.6674) knots 0 0 0 1 2 2 2
  spline S117 degree 2 poles (-54.9965, -4.6674) (-54.8038, -4.5785) (-54.2802, -4.5118) (-53.9763, -4.4945) knots 0 0 0 1 2 2 2
  line L131 (-53.9763, -4.4945) -> (-53.9763, -4.4204)
  spline S118 degree 2 poles (-53.9763, -4.4204) (-53.9763, -4.287) (-54.0579, -4.1215) (-54.132, -4.0746) knots 0 0 0 1 2 2 2
  spline S119 degree 2 poles (-54.132, -4.0746) (-54.2061, -4.0276) (-54.4185, -3.998) (-54.5321, -3.998) knots 0 0 0 1 2 2 2
  spline S120 degree 2 poles (-54.5321, -3.998) (-54.6655, -3.998) (-55.0261, -4.077) (-55.2064, -4.1536) knots 0 0 0 1 2 2 2
  line L132 (-55.2064, -4.1536) -> (-55.2286, -4.1536)
  line L133 (-55.2286, -4.1536) -> (-55.2286, -3.7609)
  spline S121 degree 2 poles (-55.2286, -3.7609) (-55.1224, -3.7312) (-54.7248, -3.6571) (-54.5296, -3.6571) knots 0 0 0 1 2 2 2
  spline S122 degree 2 poles (-54.5296, -3.6571) (-54.2925, -3.6571) (-53.9689, -3.7312) (-53.8405, -3.8276) knots 0 0 0 1 2 2 2
  spline S123 degree 2 poles (-53.8405, -3.8276) (-53.7145, -3.9214) (-53.591, -4.2203) (-53.591, -4.4352) knots 0 0 0 1 2 2 2
  line L134 (-53.591, -4.4352) -> (-53.591, -5.9987)
  line L135 (-53.591, -5.9987) -> (-53.9763, -5.9987)
  line L136 (-53.9763, -5.9987) -> (-53.9763, -5.7567)
  line L137 (-53.9763, -5.4356) -> (-53.9763, -4.8008)
  spline S124 degree 2 poles (-53.9763, -4.8008) (-54.1147, -4.8131) (-54.5321, -4.8551) (-54.663, -4.8946) knots 0 0 0 1 2 2 2
  spline S125 degree 2 poles (-54.663, -4.8946) (-54.8161, -4.9416) (-55.0162, -5.1367) (-55.0162, -5.3096) knots 0 0 0 1 2 2 2
  spline S126 degree 2 poles (-55.0162, -5.3096) (-55.0162, -5.5072) (-54.7939, -5.7073) (-54.5815, -5.7073) knots 0 0 0 1 2 2 2
  spline S127 degree 2 poles (-54.5815, -5.7073) (-54.4012, -5.7073) (-54.1048, -5.5516) (-53.9763, -5.4356) knots 0 0 0 1 2 2 2
  line L138 (-51.2914, -5.9987) -> (-51.6768, -5.9987)
  line L139 (-51.6768, -5.9987) -> (-51.6768, -5.7665)
  spline S128 degree 2 poles (-51.6768, -5.7665) (-51.7657, -5.8406) (-51.8966, -5.9394) (-51.9855, -5.9814) knots 0 0 0 1 2 2 2
  spline S129 degree 2 poles (-51.9855, -5.9814) (-52.067, -6.0209) (-52.2424, -6.0629) (-52.3585, -6.0629) knots 0 0 0 1 2 2 2
  spline S130 degree 2 poles (-52.3585, -6.0629) (-52.5462, -6.0629) (-52.8624, -5.9073) (-52.9735, -5.7567) knots 0 0 0 1 2 2 2
  spline S131 degree 2 poles (-52.9735, -5.7567) (-53.0847, -5.606) (-53.2082, -5.1614) (-53.2082, -4.8724) knots 0 0 0 1 2 2 2
  spline S132 degree 2 poles (-53.2082, -4.8724) (-53.2082, -4.5711) (-53.0526, -4.1314) (-52.9167, -3.9659) knots 0 0 0 1 2 2 2
  spline S133 degree 2 poles (-52.9167, -3.9659) (-52.7907, -3.8177) (-52.4375, -3.6473) (-52.2424, -3.6473) knots 0 0 0 1 2 2 2
  spline S134 degree 2 poles (-52.2424, -3.6473) (-52.072, -3.6473) (-51.8175, -3.7238) (-51.6768, -3.8029) knots 0 0 0 1 2 2 2
  line L140 (-51.6768, -3.8029) -> (-51.6768, -2.8149)
  line L141 (-51.6768, -2.8149) -> (-51.2914, -2.8149)
  line L142 (-51.2914, -2.8149) -> (-51.2914, -5.9987)
  line L143 (-51.6768, -5.443) -> (-51.6768, -4.1215)
  spline S135 degree 2 poles (-51.6768, -4.1215) (-51.82, -4.0523) (-52.0473, -4.0005) (-52.1782, -4.0005) knots 0 0 0 1 2 2 2
  spline S136 degree 2 poles (-52.1782, -4.0005) (-52.4746, -4.0005) (-52.8105, -4.4451) (-52.8105, -4.865) knots 0 0 0 1 2 2 2
  spline S137 degree 2 poles (-52.8105, -4.865) (-52.8105, -5.2701) (-52.5536, -5.6974) (-52.2696, -5.6974) knots 0 0 0 1 2 2 2
  spline S138 degree 2 poles (-52.2696, -5.6974) (-52.1189, -5.6974) (-51.8126, -5.5591) (-51.6768, -5.443) knots 0 0 0 1 2 2 2
  spline S139 degree 2 poles (-49.4587, -5.7567) (-49.5056, -5.7912) (-49.6637, -5.9147) (-49.7378, -5.9518) knots 0 0 0 1 2 2 2
  spline S140 degree 2 poles (-49.7378, -5.9518) (-49.8391, -6.0061) (-50.0293, -6.0629) (-50.2022, -6.0629) knots 0 0 0 1 2 2 2
  spline S141 degree 2 poles (-50.2022, -6.0629) (-50.3429, -6.0629) (-50.5974, -5.9567) (-50.6937, -5.8604) knots 0 0 0 1 2 2 2
  spline S142 degree 2 poles (-50.6937, -5.8604) (-50.7851, -5.7665) (-50.8962, -5.4899) (-50.8962, -5.3368) knots 0 0 0 1 2 2 2
  spline S143 degree 2 poles (-50.8962, -5.3368) (-50.8962, -5.0996) (-50.6962, -4.7637) (-50.4788, -4.6674) knots 0 0 0 1 2 2 2
  spline S144 degree 2 poles (-50.4788, -4.6674) (-50.2861, -4.5785) (-49.7625, -4.5118) (-49.4587, -4.4945) knots 0 0 0 1 2 2 2
  line L144 (-49.4587, -4.4945) -> (-49.4587, -4.4204)
  spline S145 degree 2 poles (-49.4587, -4.4204) (-49.4587, -4.287) (-49.5402, -4.1215) (-49.6143, -4.0746) knots 0 0 0 1 2 2 2
  spline S146 degree 2 poles (-49.6143, -4.0746) (-49.6884, -4.0276) (-49.9008, -3.998) (-50.0144, -3.998) knots 0 0 0 1 2 2 2
  spline S147 degree 2 poles (-50.0144, -3.998) (-50.1478, -3.998) (-50.5084, -4.077) (-50.6888, -4.1536) knots 0 0 0 1 2 2 2
  line L145 (-50.6888, -4.1536) -> (-50.711, -4.1536)
  line L146 (-50.711, -4.1536) -> (-50.711, -3.7609)
  spline S148 degree 2 poles (-50.711, -3.7609) (-50.6048, -3.7312) (-50.2071, -3.6571) (-50.012, -3.6571) knots 0 0 0 1 2 2 2
  spline S149 degree 2 poles (-50.012, -3.6571) (-49.7748, -3.6571) (-49.4513, -3.7312) (-49.3228, -3.8276) knots 0 0 0 1 2 2 2
  spline S150 degree 2 poles (-49.3228, -3.8276) (-49.1969, -3.9214) (-49.0734, -4.2203) (-49.0734, -4.4352) knots 0 0 0 1 2 2 2
  line L147 (-49.0734, -4.4352) -> (-49.0734, -5.9987)
  line L148 (-49.0734, -5.9987) -> (-49.4587, -5.9987)
  line L149 (-49.4587, -5.9987) -> (-49.4587, -5.7567)
  line L150 (-49.4587, -5.4356) -> (-49.4587, -4.8008)
  spline S151 degree 2 poles (-49.4587, -4.8008) (-49.597, -4.8131) (-50.0144, -4.8551) (-50.1453, -4.8946) knots 0 0 0 1 2 2 2
  spline S152 degree 2 poles (-50.1453, -4.8946) (-50.2985, -4.9416) (-50.4986, -5.1367) (-50.4986, -5.3096) knots 0 0 0 1 2 2 2
  spline S153 degree 2 poles (-50.4986, -5.3096) (-50.4986, -5.5072) (-50.2763, -5.7073) (-50.0638, -5.7073) knots 0 0 0 1 2 2 2
  spline S154 degree 2 poles (-50.0638, -5.7073) (-49.8835, -5.7073) (-49.5871, -5.5516) (-49.4587, -5.4356) knots 0 0 0 1 2 2 2
  line L151 (-48.1397, -5.9987) -> (-48.525, -5.9987)
  line L152 (-48.525, -5.9987) -> (-48.525, -2.8149)
  line L153 (-48.525, -2.8149) -> (-48.1397, -2.8149)
  line L154 (-48.1397, -2.8149) -> (-48.1397, -5.9987)
  spline S155 degree 2 poles (-46.2995, -5.7567) (-46.3465, -5.7912) (-46.5045, -5.9147) (-46.5786, -5.9518) knots 0 0 0 1 2 2 2
  spline S156 degree 2 poles (-46.5786, -5.9518) (-46.6799, -6.0061) (-46.8701, -6.0629) (-47.043, -6.0629) knots 0 0 0 1 2 2 2
  spline S157 degree 2 poles (-47.043, -6.0629) (-47.1838, -6.0629) (-47.4382, -5.9567) (-47.5345, -5.8604) knots 0 0 0 1 2 2 2
  spline S158 degree 2 poles (-47.5345, -5.8604) (-47.6259, -5.7665) (-47.7371, -5.4899) (-47.7371, -5.3368) knots 0 0 0 1 2 2 2
  spline S159 degree 2 poles (-47.7371, -5.3368) (-47.7371, -5.0996) (-47.537, -4.7637) (-47.3196, -4.6674) knots 0 0 0 1 2 2 2
  spline S160 degree 2 poles (-47.3196, -4.6674) (-47.127, -4.5785) (-46.6033, -4.5118) (-46.2995, -4.4945) knots 0 0 0 1 2 2 2
  line L155 (-46.2995, -4.4945) -> (-46.2995, -4.4204)
  spline S161 degree 2 poles (-46.2995, -4.4204) (-46.2995, -4.287) (-46.381, -4.1215) (-46.4551, -4.0746) knots 0 0 0 1 2 2 2
  spline S162 degree 2 poles (-46.4551, -4.0746) (-46.5292, -4.0276) (-46.7417, -3.998) (-46.8553, -3.998) knots 0 0 0 1 2 2 2
  spline S163 degree 2 poles (-46.8553, -3.998) (-46.9887, -3.998) (-47.3493, -4.077) (-47.5296, -4.1536) knots 0 0 0 1 2 2 2
  line L156 (-47.5296, -4.1536) -> (-47.5518, -4.1536)
  line L157 (-47.5518, -4.1536) -> (-47.5518, -3.7609)
  spline S164 degree 2 poles (-47.5518, -3.7609) (-47.4456, -3.7312) (-47.0479, -3.6571) (-46.8528, -3.6571) knots 0 0 0 1 2 2 2
  spline S165 degree 2 poles (-46.8528, -3.6571) (-46.6157, -3.6571) (-46.2921, -3.7312) (-46.1637, -3.8276) knots 0 0 0 1 2 2 2
  spline S166 degree 2 poles (-46.1637, -3.8276) (-46.0377, -3.9214) (-45.9142, -4.2203) (-45.9142, -4.4352) knots 0 0 0 1 2 2 2
  line L158 (-45.9142, -4.4352) -> (-45.9142, -5.9987)
  line L159 (-45.9142, -5.9987) -> (-46.2995, -5.9987)
  line L160 (-46.2995, -5.9987) -> (-46.2995, -5.7567)
  line L161 (-46.2995, -5.4356) -> (-46.2995, -4.8008)
  spline S167 degree 2 poles (-46.2995, -4.8008) (-46.4379, -4.8131) (-46.8553, -4.8551) (-46.9862, -4.8946) knots 0 0 0 1 2 2 2
  spline S168 degree 2 poles (-46.9862, -4.8946) (-47.1393, -4.9416) (-47.3394, -5.1367) (-47.3394, -5.3096) knots 0 0 0 1 2 2 2
  spline S169 degree 2 poles (-47.3394, -5.3096) (-47.3394, -5.5072) (-47.1171, -5.7073) (-46.9047, -5.7073) knots 0 0 0 1 2 2 2
  spline S170 degree 2 poles (-46.9047, -5.7073) (-46.7244, -5.7073) (-46.428, -5.5516) (-46.2995, -5.4356) knots 0 0 0 1 2 2 2
  line L162 (-42.7798, -5.9987) -> (-42.7798, -4.6748)
  spline S171 degree 2 poles (-42.7798, -4.6748) (-42.7798, -4.5167) (-42.8045, -4.2475) (-42.844, -4.1734) knots 0 0 0 1 2 2 2
  spline S172 degree 2 poles (-42.844, -4.1734) (-42.8835, -4.0919) (-43.0342, -4.0128) (-43.1651, -4.0128) knots 0 0 0 1 2 2 2
  spline S173 degree 2 poles (-43.1651, -4.0128) (-43.2836, -4.0128) (-43.5553, -4.1586) (-43.6986, -4.2969) knots 0 0 0 1 2 2 2
  spline S174 degree 2 poles (-43.6986, -4.2969) (-43.6961, -4.3315) (-43.6912, -4.4278) (-43.6912, -4.492) knots 0 0 0 1 2 2 2
  line L163 (-43.6912, -4.492) -> (-43.6912, -5.9987)
  line L164 (-43.6912, -5.9987) -> (-44.0765, -5.9987)
  line L165 (-44.0765, -5.9987) -> (-44.0765, -4.6748)
  spline S175 degree 2 poles (-44.0765, -4.6748) (-44.0765, -4.5167) (-44.1012, -4.2475) (-44.1407, -4.1734) knots 0 0 0 1 2 2 2
  spline S176 degree 2 poles (-44.1407, -4.1734) (-44.1803, -4.0919) (-44.3309, -4.0128) (-44.4618, -4.0128) knots 0 0 0 1 2 2 2
  spline S177 degree 2 poles (-44.4618, -4.0128) (-44.5853, -4.0128) (-44.8595, -4.1684) (-44.988, -4.2895) knots 0 0 0 1 2 2 2
  line L166 (-44.988, -4.2895) -> (-44.988, -5.9987)
  line L167 (-44.988, -5.9987) -> (-45.3733, -5.9987)
  line L168 (-45.3733, -5.9987) -> (-45.3733, -3.7115)
  line L169 (-45.3733, -3.7115) -> (-44.988, -3.7115)
  line L170 (-44.988, -3.7115) -> (-44.988, -3.9634)
  spline S178 degree 2 poles (-44.988, -3.9634) (-44.8373, -3.8128) (-44.5409, -3.6473) (-44.363, -3.6473) knots 0 0 0 1 2 2 2
  spline S179 degree 2 poles (-44.363, -3.6473) (-44.1605, -3.6473) (-43.8468, -3.8325) (-43.7653, -4.0425) knots 0 0 0 1 2 2 2
  spline S180 degree 2 poles (-43.7653, -4.0425) (-43.5899, -3.8473) (-43.2589, -3.6473) (-43.0663, -3.6473) knots 0 0 0 1 2 2 2
  spline S181 degree 2 poles (-43.0663, -3.6473) (-42.9181, -3.6473) (-42.676, -3.7387) (-42.5871, -3.8424) knots 0 0 0 1 2 2 2
  spline S182 degree 2 poles (-42.5871, -3.8424) (-42.4957, -3.9461) (-42.3944, -4.2574) (-42.3944, -4.492) knots 0 0 0 1 2 2 2
  line L171 (-42.3944, -4.492) -> (-42.3944, -5.9987)
  line L172 (-42.3944, -5.9987) -> (-42.7798, -5.9987)
  spline S183 degree 2 poles (-40.8606, -6.0506) (-41.4089, -6.0506) (-42.0116, -5.4356) (-42.0116, -4.8675) knots 0 0 0 1 2 2 2
  spline S184 degree 2 poles (-42.0116, -4.8675) (-42.0116, -4.3092) (-41.4262, -3.6473) (-40.9544, -3.6473) knots 0 0 0 1 2 2 2
  spline S185 degree 2 poles (-40.9544, -3.6473) (-40.742, -3.6473) (-40.4135, -3.7708) (-40.2925, -3.9017) knots 0 0 0 1 2 2 2
  spline S186 degree 2 poles (-40.2925, -3.9017) (-40.169, -4.0326) (-40.038, -4.4105) (-40.038, -4.6847) knots 0 0 0 1 2 2 2
  line L173 (-40.038, -4.6847) -> (-40.038, -4.8946)
  line L174 (-40.038, -4.8946) -> (-41.6213, -4.8946)
  spline S187 degree 2 poles (-41.6213, -4.8946) (-41.6213, -5.2923) (-41.2212, -5.7147) (-40.8655, -5.7147) knots 0 0 0 1 2 2 2
  spline S188 degree 2 poles (-40.8655, -5.7147) (-40.7395, -5.7147) (-40.495, -5.6579) (-40.3962, -5.6134) knots 0 0 0 1 2 2 2
  spline S189 degree 2 poles (-40.3962, -5.6134) (-40.2925, -5.564) (-40.1492, -5.4775) (-40.1023, -5.438) knots 0 0 0 1 2 2 2
  line L175 (-40.1023, -5.438) -> (-40.08, -5.438)
  line L176 (-40.08, -5.438) -> (-40.08, -5.8579)
  spline S190 degree 2 poles (-40.08, -5.8579) (-40.1467, -5.8851) (-40.3493, -5.9641) (-40.4283, -5.9864) knots 0 0 0 1 2 2 2
  spline S191 degree 2 poles (-40.4283, -5.9864) (-40.5395, -6.0185) (-40.7222, -6.0506) (-40.8606, -6.0506) knots 0 0 0 1 2 2 2
  spline S192 degree 2 poles (-40.4135, -4.6007) (-40.4184, -4.4451) (-40.4826, -4.2178) (-40.5444, -4.1413) knots 0 0 0 1 2 2 2
  spline S193 degree 2 poles (-40.5444, -4.1413) (-40.6111, -4.0548) (-40.821, -3.9634) (-40.9766, -3.9634) knots 0 0 0 1 2 2 2
  spline S194 degree 2 poles (-40.9766, -3.9634) (-41.1298, -3.9634) (-41.3447, -4.0548) (-41.4336, -4.1437) knots 0 0 0 1 2 2 2
  spline S195 degree 2 poles (-41.4336, -4.1437) (-41.5201, -4.2351) (-41.609, -4.455) (-41.6213, -4.6007) knots 0 0 0 1 2 2 2
  line L177 (-41.6213, -4.6007) -> (-40.4135, -4.6007)
  line L178 (-37.8521, -5.9987) -> (-38.2374, -5.9987)
  line L179 (-38.2374, -5.9987) -> (-38.2374, -4.6946)
  spline S196 degree 2 poles (-38.2374, -4.6946) (-38.2374, -4.5365) (-38.267, -4.2648) (-38.3115, -4.1833) knots 0 0 0 1 2 2 2
  spline S197 degree 2 poles (-38.3115, -4.1833) (-38.3584, -4.0968) (-38.5264, -4.0128) (-38.6697, -4.0128) knots 0 0 0 1 2 2 2
  spline S198 degree 2 poles (-38.6697, -4.0128) (-38.8129, -4.0128) (-39.1167, -4.166) (-39.2625, -4.2895) knots 0 0 0 1 2 2 2
  line L180 (-39.2625, -4.2895) -> (-39.2625, -5.9987)
  line L181 (-39.2625, -5.9987) -> (-39.6478, -5.9987)
  line L182 (-39.6478, -5.9987) -> (-39.6478, -3.7115)
  line L183 (-39.6478, -3.7115) -> (-39.2625, -3.7115)
  line L184 (-39.2625, -3.7115) -> (-39.2625, -3.9659)
  spline S199 degree 2 poles (-39.2625, -3.9659) (-39.0896, -3.8103) (-38.7561, -3.6473) (-38.5684, -3.6473) knots 0 0 0 1 2 2 2
  spline S200 degree 2 poles (-38.5684, -3.6473) (-38.2325, -3.6473) (-37.8521, -4.0919) (-37.8521, -4.5142) knots 0 0 0 1 2 2 2
  line L185 (-37.8521, -4.5142) -> (-37.8521, -5.9987)
  spline S201 degree 2 poles (-36.6195, -6.0432) (-36.9332, -6.0432) (-37.2864, -5.685) (-37.2864, -5.2972) knots 0 0 0 1 2 2 2
  line L186 (-37.2864, -5.2972) -> (-37.2864, -4.0301)
  line L187 (-37.2864, -4.0301) -> (-37.5458, -4.0301)
  line L188 (-37.5458, -4.0301) -> (-37.5458, -3.7115)
  line L189 (-37.5458, -3.7115) -> (-37.2864, -3.7115)
  line L190 (-37.2864, -3.7115) -> (-37.2864, -3.0545)
  line L191 (-37.2864, -3.0545) -> (-36.9011, -3.0545)
  line L192 (-36.9011, -3.0545) -> (-36.9011, -3.7115)
  line L193 (-36.9011, -3.7115) -> (-36.1922, -3.7115)
  line L194 (-36.1922, -3.7115) -> (-36.1922, -4.0301)
  line L195 (-36.1922, -4.0301) -> (-36.9011, -4.0301)
  line L196 (-36.9011, -4.0301) -> (-36.9011, -5.1194)
  spline S202 degree 2 poles (-36.9011, -5.1194) (-36.9011, -5.2923) (-36.8888, -5.4825) (-36.8468, -5.564) knots 0 0 0 1 2 2 2
  spline S203 degree 2 poles (-36.8468, -5.564) (-36.8122, -5.6356) (-36.6566, -5.7073) (-36.5232, -5.7073) knots 0 0 0 1 2 2 2
  spline S204 degree 2 poles (-36.5232, -5.7073) (-36.4293, -5.7073) (-36.254, -5.6504) (-36.2145, -5.6332) knots 0 0 0 1 2 2 2
  line L197 (-36.2145, -5.6332) -> (-36.1922, -5.6332)
  line L198 (-36.1922, -5.6332) -> (-36.1922, -5.979)
  spline S205 degree 2 poles (-36.1922, -5.979) (-36.3009, -6.0086) (-36.5232, -6.0432) (-36.6195, -6.0432) knots 0 0 0 1 2 2 2
  line L199 (-35.5154, -5.9987) -> (-35.9008, -5.9987)
  line L200 (-35.9008, -5.9987) -> (-35.9008, -3.7115)
  line L201 (-35.9008, -3.7115) -> (-35.5154, -3.7115)
  line L202 (-35.5154, -3.7115) -> (-35.5154, -5.9987)
  line L203 (-35.4883, -3.3311) -> (-35.9255, -3.3311)
  line L204 (-35.9255, -3.3311) -> (-35.9255, -2.931)
  line L205 (-35.9255, -2.931) -> (-35.4883, -2.931)
  line L206 (-35.4883, -2.931) -> (-35.4883, -3.3311)
  line L207 (-31.7882, -3.3113) -> (-33.206, -3.3113)
  line L208 (-33.206, -3.3113) -> (-33.206, -4.1709)
  line L209 (-33.206, -4.1709) -> (-31.8475, -4.1709)
  line L210 (-31.8475, -4.1709) -> (-31.8475, -4.5315)
  line L211 (-31.8475, -4.5315) -> (-33.206, -4.5315)
  line L212 (-33.206, -4.5315) -> (-33.206, -5.9987)
  line L213 (-33.206, -5.9987) -> (-33.6111, -5.9987)
  line L214 (-33.6111, -5.9987) -> (-33.6111, -2.9507)
  line L215 (-33.6111, -2.9507) -> (-31.7882, -2.9507)
  line L216 (-31.7882, -2.9507) -> (-31.7882, -3.3113)
  line L217 (-31.062, -5.9987) -> (-31.4473, -5.9987)
  line L218 (-31.4473, -5.9987) -> (-31.4473, -3.7115)
  line L219 (-31.4473, -3.7115) -> (-31.062, -3.7115)
  line L220 (-31.062, -3.7115) -> (-31.062, -5.9987)
  line L221 (-31.0348, -3.3311) -> (-31.472, -3.3311)
  line L222 (-31.472, -3.3311) -> (-31.472, -2.931)
  line L223 (-31.472, -2.931) -> (-31.0348, -2.931)
  line L224 (-31.0348, -2.931) -> (-31.0348, -3.3311)
  line L225 (-30.1036, -5.9987) -> (-30.489, -5.9987)
  line L226 (-30.489, -5.9987) -> (-30.489, -2.8149)
  line L227 (-30.489, -2.8149) -> (-30.1036, -2.8149)
  line L228 (-30.1036, -2.8149) -> (-30.1036, -5.9987)
  line L229 (-29.1453, -5.9987) -> (-29.5306, -5.9987)
  line L230 (-29.5306, -5.9987) -> (-29.5306, -3.7115)
  line L231 (-29.5306, -3.7115) -> (-29.1453, -3.7115)
  line L232 (-29.1453, -3.7115) -> (-29.1453, -5.9987)
  line L233 (-29.1181, -3.3311) -> (-29.5553, -3.3311)
  line L234 (-29.5553, -3.3311) -> (-29.5553, -2.931)
  line L235 (-29.5553, -2.931) -> (-29.1181, -2.931)
  line L236 (-29.1181, -2.931) -> (-29.1181, -3.3311)
  spline S206 degree 2 poles (-26.6629, -4.7934) (-26.6629, -5.3664) (-27.2088, -6.0432) (-27.6262, -6.0432) knots 0 0 0 1 2 2 2
  spline S207 degree 2 poles (-27.6262, -6.0432) (-27.7966, -6.0432) (-28.0585, -5.9641) (-28.1943, -5.8826) knots 0 0 0 1 2 2 2
  line L237 (-28.1943, -5.8826) -> (-28.1943, -6.841)
  line L238 (-28.1943, -6.841) -> (-28.5796, -6.841)
  line L239 (-28.5796, -6.841) -> (-28.5796, -3.7115)
  line L240 (-28.5796, -3.7115) -> (-28.1943, -3.7115)
  line L241 (-28.1943, -3.7115) -> (-28.1943, -3.9511)
  spline S208 degree 2 poles (-28.1943, -3.9511) (-28.0511, -3.8202) (-27.7003, -3.6473) (-27.4953, -3.6473) knots 0 0 0 1 2 2 2
  spline S209 degree 2 poles (-27.4953, -3.6473) (-27.1026, -3.6473) (-26.6629, -4.2697) (-26.6629, -4.7934) knots 0 0 0 1 2 2 2
  spline S210 degree 2 poles (-27.0606, -4.8378) (-27.0606, -4.4451) (-27.31, -4.0128) (-27.5892, -4.0128) knots 0 0 0 1 2 2 2
  spline S211 degree 2 poles (-27.5892, -4.0128) (-27.7522, -4.0128) (-28.0585, -4.1586) (-28.1943, -4.2722) knots 0 0 0 1 2 2 2
  line L242 (-28.1943, -4.2722) -> (-28.1943, -5.5714)
  spline S212 degree 2 poles (-28.1943, -5.5714) (-28.0436, -5.643) (-27.8288, -5.6974) (-27.6904, -5.6974) knots 0 0 0 1 2 2 2
  spline S213 degree 2 poles (-27.6904, -5.6974) (-27.3916, -5.6974) (-27.0606, -5.2577) (-27.0606, -4.8378) knots 0 0 0 1 2 2 2
  spline S214 degree 2 poles (-24.346, -4.7934) (-24.346, -5.3664) (-24.8919, -6.0432) (-25.3093, -6.0432) knots 0 0 0 1 2 2 2
  spline S215 degree 2 poles (-25.3093, -6.0432) (-25.4798, -6.0432) (-25.7416, -5.9641) (-25.8774, -5.8826) knots 0 0 0 1 2 2 2
  line L243 (-25.8774, -5.8826) -> (-25.8774, -6.841)
  line L244 (-25.8774, -6.841) -> (-26.2628, -6.841)
  line L245 (-26.2628, -6.841) -> (-26.2628, -3.7115)
  line L246 (-26.2628, -3.7115) -> (-25.8774, -3.7115)
  line L247 (-25.8774, -3.7115) -> (-25.8774, -3.9511)
  spline S216 degree 2 poles (-25.8774, -3.9511) (-25.7342, -3.8202) (-25.3834, -3.6473) (-25.1784, -3.6473) knots 0 0 0 1 2 2 2
  spline S217 degree 2 poles (-25.1784, -3.6473) (-24.7857, -3.6473) (-24.346, -4.2697) (-24.346, -4.7934) knots 0 0 0 1 2 2 2
  spline S218 degree 2 poles (-24.7437, -4.8378) (-24.7437, -4.4451) (-24.9932, -4.0128) (-25.2723, -4.0128) knots 0 0 0 1 2 2 2
  spline S219 degree 2 poles (-25.2723, -4.0128) (-25.4353, -4.0128) (-25.7416, -4.1586) (-25.8774, -4.2722) knots 0 0 0 1 2 2 2
  line L248 (-25.8774, -4.2722) -> (-25.8774, -5.5714)
  spline S220 degree 2 poles (-25.8774, -5.5714) (-25.7268, -5.643) (-25.5119, -5.6974) (-25.3736, -5.6974) knots 0 0 0 1 2 2 2
  spline S221 degree 2 poles (-25.3736, -5.6974) (-25.0747, -5.6974) (-24.7437, -5.2577) (-24.7437, -4.8378) knots 0 0 0 1 2 2 2
  spline S222 degree 2 poles (-22.0662, -4.8551) (-22.0662, -5.4331) (-22.622, -6.0629) (-23.0863, -6.0629) knots 0 0 0 1 2 2 2
  spline S223 degree 2 poles (-23.0863, -6.0629) (-23.563, -6.0629) (-24.1089, -5.4133) (-24.1089, -4.8551) knots 0 0 0 1 2 2 2
  spline S224 degree 2 poles (-24.1089, -4.8551) (-24.1089, -4.2821) (-23.5457, -3.6473) (-23.0863, -3.6473) knots 0 0 0 1 2 2 2